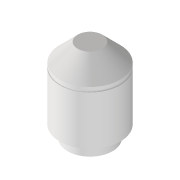
# Autodesk Inventor part: 00_10x_Objective_ViewSolutions_bm05073332
Saved by Autodesk Inventor 2022 (Build 260153000, 153)
## iProperties
Created: 2023-01-02
Part Number: 00_10x_Objective_ViewSolutions_bm05073332
Material: Generisch
Document SubType Name: Modeling
Designer: diederichbenedict
Density: 1 g/cm^3
Appearance: Vorgabe
Author: diederichbenedict
Autodesk Inventor part; units mm, degrees
ref_plane "YZ Plane" through (0, 0, 0) normal (1, 0, 0) x (0, 1, 0)
ref_plane "XZ Plane" through (0, 0, 0) normal (0, 1, 0) x (-1, 0, 0)
ref_plane "XY Plane" through (0, 0, 0) normal (0, 0, 1) x (1, 0, 0)
sketch "Skizze1" plane through (0, 0, 0) normal (1, 0, 0) x (0, 1, 0)
  line L0 (0, 13.5) -> (24, 13.5)
  line L1 (24, 13.5) -> (32, 5.5)
  line L2 (32, 5.5) -> (32, 0)
  line L3 (32, 0) -> (0, 0)
  line L4 (0, 0) -> (0, 13.5)
  arc A0 (21.85, 13.5) -> (22.85, 13.5) centre (22.35, 13.5) ccw
  line L5 (0, 0) -> (-0.5, 0)
  line L6 (-0.5, 0) -> (-0.5, 12.225)
  line L7 (-0.5, 12.225) -> (0, 12.225)
  line L8 (0, 12.225) -> (0, 0)
  line L9 (-0.5, 0) -> (-5.43, 0)
  line L10 (-5.43, 0) -> (-5.43, 10.08)
  line L11 (-5.43, 10.08) -> (-0.5, 10.08)
  line L12 (-0.5, 10.08) -> (-0.5, 0)
  point P0 (-0.5, 10.08)
  dimension "d0" = 24
  dimension "d1" = 135
  dimension "d2" = 5.5
  dimension "d3" = 1
  dimension "d4" = 0.5
  dimension "d5" = 1.15
  dimension "d6" = 0.5
  dimension "d7" = 12.225
  dimension "d8" = 4.93
  dimension "d9" = 10.08
  constraints: 26 end point, 5 perpendicular, 4 parallel, 3 horizontal, 2 point on circle, 2 point on line, 1 centre point
  measures "d0" distance of L0.start L0.end
  measures "d1" angle of L0 L1
  measures "d2" distance of L2.end L1.end
  measures "d3" distance of A0.start A0.end
  measures "d4" radius of A0
  measures "d5" distance of A0.end L0.end
  measures "d6" distance of L6.end L7.end
  measures "d7" distance of L5.end L6.end
  measures "d8" distance of L10.end L11.end
  measures "d9" distance of L9.end L10.end
revolve "Umdrehung1" add sketch "Skizze1" angle 360 about axis through (0, 32, 0) along (0, -1, 0) contours L0 A0 L1 L2 L3 L4 | L4 L5 L6 L7 | L9 L10 L11 L6
